Batterie Holder (Autodesk Fusion 360 design; units mm, degrees)
Autodesk Fusion 360 part; units mm, degrees
sketch "Sketch1" plane through (0, 0, 0) normal (0, 1, 0) x (1, 0, 0)
  circle A0 centre (0, 0) radius 2.95
  line L0 (0, 0) -> (25, 0) construction
  line L1 (25, -32.2093) -> (25, 32.2093)
  circle A1 centre (0, 0) radius 5
  line L2 (0, 5) -> (25, 5)
  line L3 (5, 0) -> (25, 0)
  line L4 (16.25, 0) -> (16.25, -5)
  line L5 (16.25, -5) -> (11.25, -5)
  line L6 (11.25, -5) -> (6.25, 0)
  line L7 (11.25, -5) -> (18.3211, -5) construction
  dimension "d1" = 5.9
  dimension "d2" = 25
  dimension "d3" = 10
  dimension "d4" = 17.5
  dimension "d5" = 5
  dimension "d6" = 5
  dimension "d7" = 135
  constraint coincident A0.centre L0.start
  constraint horizontal L0
  constraint vertical L1
  constraint midpoint L0.end L1
  constraint concentric A0 A1
  constraint coincident A1 L2.start
  constraint coincident L1 L2.end
  constraint tangent A1 L2
  constraint perpendicular L1 L2
  constraint coincident L0 L3.start
  constraint coincident A1 L3.start
  constraint coincident L0 L4.start
  constraint perpendicular L0 L4
  constraint perpendicular L4 L5
  constraint horizontal L7
  constraint coincident L3 L6.end
  measures "d1" diameter of A0
  measures "d2" distance of A0.centre L0.end
  measures "d3" diameter of A1
  measures "d5" distance of L4.start L4.end
  measures "d6" distance of L4.end L5.end
  measures "d7" angle of L6 L7
extrude "Extrude1" add sketch "Sketch1" along normal blind 5
sketch "Sketch2" plane through (0, 0, 0) normal (0, -1, 0) x (1, 0, 0)
  circle A0 centre (0, 0) radius 2.95
  line L0 (25, 0) -> (16.25, 0)
  line L1 (16.25, 0) -> (16.25, 5)
  line L2 (16.25, 5) -> (11.25, 5)
  line L3 (11.25, 5) -> (6.25, 0)
  line L4 (6.25, 0) -> (5, 0)
  arc A1 (5, 0) -> (0, -5) centre (0, 0) ccw
  line L5 (0, -5) -> (25, -5)
  line L6 (25, -5) -> (25, 0)
  line L7 (6.25, 0) -> (6.25, -5)
  constraint coincident L3.end L4.start
  constraint coincident L5 L7.end
  constraint perpendicular L5 L7
extrude "Extrude2" add sketch "Sketch2" along normal blind 20 contours L0 L1 L2 L3 L5 L6 L7
sketch "Sketch3" plane through (0, -20, 0) normal (0, -1, 0) x (1, 0, 0)
  line L0 (6.25, 0) -> (6.25, -5)
  line L1 (6.25, -5) -> (25, -5)
  line L2 (25, -5) -> (25, 0)
  line L3 (25, 0) -> (16.25, 0)
  line L4 (16.25, 0) -> (16.25, 5)
  line L5 (16.25, 5) -> (11.25, 5)
  line L6 (11.25, 5) -> (6.25, 0)
  line L7 (6.25, -5) -> (6.25, 0)
  line L8 (6.25, 0) -> (5, 0)
  arc A0 (5, 0) -> (0, -5) centre (0, 0) ccw
  line L9 (0, -5) -> (6.25, -5)
  circle A1 centre (0, 0) radius 2.95
extrude "Extrude3" add sketch "Sketch3" along normal blind 5
mirror "Mirror1" about plane through (25, -20, -5) normal (1, 0, 0) of bodies 1 merged
sketch "Sketch4" plane through (0, 0, 0) normal (0, 0, 1) x (-1, 0, 0)
  line L0 (-33.75, -5) -> (-16.25, -5)
  line L1 (-16.25, -5) -> (-16.25, 25)
  line L2 (-16.25, 25) -> (-33.75, 25)
  line L3 (-33.75, 25) -> (-33.75, -5)
  line L4 (-33.75, 25) -> (-16.25, 25)
  line L5 (-16.25, 25) -> (-16.25, 20)
  line L6 (-16.25, 20) -> (-33.75, 20)
  line L7 (-33.75, 20) -> (-33.75, 25)
  dimension "d16" = 17.5
  dimension "d17" = 5
  constraint horizontal L4
  constraint vertical L5
  constraint horizontal L6
  constraint vertical L7
  constraint coincident L2.end L3.start
  measures "d16" distance of L2.end L1.end
  measures "d17" distance of L2.end L6.end
extrude "Extrude4" cut sketch "Sketch4" against normal blind 5 contours L1 L2 L3 L4 L5 L6 L7
extrude "Extrude5" cut 2 faces at (11.25, -25, 0) (38.75, -25, 0) along direction (0, 1, 0) blind 5
